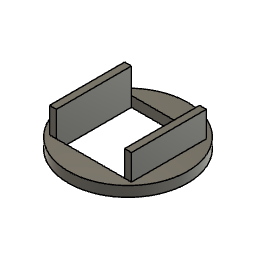
PCB Caps (Autodesk Fusion 360 design; units mm, degrees)
Autodesk Fusion 360 part; units mm, degrees
sketch "Sketch1" plane through (0, 0, 0) normal (0, 1, 0) x (1, 0, 0) in component "PCBCap"
  circle A0 centre (0, 0) radius 17.5
  dimension "d1" = 35
  constraint coincident A0.centre origin
  measures "d1" diameter of A0
extrude "Extrude1" add sketch "Sketch1" along normal blind 3 in component "PCBCap"
sketch "Sketch2" plane through (0, 3, 0) normal (0, 1, 0) x (-1, 0, 0) in component "PCBCap"
  circle A0 centre (0, 0) radius 17.5
  line L0 (12, 11) -> (12, -11)
  line L1 (-12, 11) -> (-12, -11)
  line L2 (0, 1.75) -> (0, 22.5)
  line L3 (-1.75, 0) -> (-22.5, 0)
  line L4 (12, -11) -> (10, -11)
  line L5 (10, -11) -> (10, 11)
  line L6 (10, 11) -> (12, 11)
  line L7 (12, 11) -> (12, -11)
  line L8 (-12, -11) -> (-10, -11)
  line L9 (-10, -11) -> (-10, 11)
  line L10 (-10, 11) -> (-12, 11)
  line L11 (-12, 11) -> (-12, -11)
  point P0 (12, 0)
  point P1 (-12, 0)
  dimension "d4" = 22
  dimension "d5" = 22
  dimension "d10" = 2
  dimension "d11" = 2
  dimension "d12" = 20
  constraint vertical L0
  constraint midpoint L0 P0
  constraint vertical L1
  constraint symmetric L0 L1 L2
  constraint coincident P0 L3
  constraint midpoint L1 P1
  constraint coincident L3 P1
  constraint horizontal L4
  constraint vertical L5
  constraint horizontal L6
  constraint vertical L7
  constraint horizontal L8
  constraint vertical L9
  constraint horizontal L10
  constraint vertical L11
  measures "d4" distance of L0.start L0.end
  measures "d5" distance of L1.start L1.end
  measures "d10" distance of L0.end L4.end
  measures "d11" distance of L1.end L8.end
  measures "d12" distance of L5 L9
extrude "Extrude2" add sketch "Sketch2" along normal blind 7.5 contours L0 L4 L5 L6 L7 | L1 L3 L9 L10 L11 | L1 L3 L8 L9 L11 in component "PCBCap"
sketch "Sketch3" plane through (0, 3, 0) normal (0, 1, 0) x (-1, 0, 0) in component "PCBCap"
  line L0 (-12, 11) -> (-10, 11)
  line L1 (-10, 11) -> (-10, -11)
  line L2 (-10, -11) -> (-12, -11)
  line L3 (-12, -11) -> (-12, 11)
  line L4 (12, 11) -> (12, -11)
  line L5 (12, -11) -> (10, -11)
  line L6 (10, -11) -> (10, 11)
  line L7 (10, 11) -> (12, 11)
  circle A0 centre (0, 0) radius 17.5
  line L8 (10, -11) -> (-10, -11)
  line L9 (-10, -11) -> (-10, 11)
  line L10 (-10, 11) -> (10, 11)
  line L11 (10, 11) -> (10, -11)
  constraint horizontal L8
  constraint vertical L9
  constraint horizontal L10
  constraint vertical L11
  constraint coincident L5.end L6.start
extrude "Extrude3" cut sketch "Sketch3" against normal through all contours L1 L6 L8 L9 L10 L11 in component "PCBCap"
component "PCBCap" placed x (1, 0, 0) y (0, 1, 0) z (0, 0, 1) at (0, 0, 0)
equation "d4 = PCBWidth + 2 * ( PCBWidthTolerance )"
equation "d5 = PCBWidth + 2 * ( PCBWidthTolerance )"
equation "PCBWidth = 20 mm" comment "Width of the PCB"
equation "PCBWidthTolerance = 1 mm" comment "Additional Width for PCB"
equation "PCBWallThickness = 2 mm" comment "Thickness of PCB Wall"
equation "d10 = PCBWallThickness"
equation "d11 = PCBWallThickness"
equation "d12 = PCBWallSpread"
equation "PCBWallSpread = 20 mm" comment "Distance between the two PCB Walls"
equation "PCBWallLength = 7.5 mm" comment "Length of the PCB Wall for screwing in"
